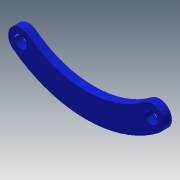
# Autodesk Inventor part: neco
Saved by Autodesk Inventor 2013 (Build 170138000, 138)
## iProperties
Created: 2013-03-09
Part Number: neco
Material: Generic
Document SubType Name: Modeling
Designer: idle-rug
Density: 1 g/cm^3
Author: idle-rug
Autodesk Inventor part; units mm, degrees
ref_plane "YZ Plane" through (0, 0, 0) normal (1, 0, 0) x (0, 1, 0)
ref_plane "XZ Plane" through (0, 0, 0) normal (0, 1, 0) x (-1, 0, 0)
ref_plane "XY Plane" through (0, 0, 0) normal (0, 0, 1) x (1, 0, 0)
sketch "Sketch1" plane through (0, 0, 0) normal (0, 1, 0) x (-1, 0, 0)
  line L0 (0, 0) -> (16, 0)
  line L1 (0, 0) -> (-16, 0)
  circle A0 centre (16, 0) radius 1.5
  circle A1 centre (-16, 0) radius 1.5
  circle A2 centre (16, 0) radius 3
  circle A3 centre (-16, 0) radius 3
  line L2 (14.1819, 2.3863) -> (16, 0)
  line L3 (16, 0) -> (17.8181, -2.3863)
  line L4 (-14.1819, 2.3863) -> (-16, 0)
  line L5 (-16, 0) -> (-17.8181, -2.3863)
  line L6 (0, -2.4008) -> (0, -8.4008)
  arc A4 (-17.8181, -2.3863) -> (17.8181, -2.3863) centre (0, 21) ccw
  arc A5 (-14.1819, 2.3863) -> (14.1819, 2.3863) centre (0, 21) ccw
  dimension "d2" = 3
  dimension "d11" = 6
  constraints: 14 end point, 10 point on circle, 6 centre point, 4 coincident, 3 collinear, 1 horizontal
  measures "d2" diameter of A0
  measures "d11" distance of L6.start L6.end
extrude "Extrusion1" add sketch "Sketch1" along normal blind 2 contours A5 A2 L0 | L0 A2 A4 L6 A5 | A5 L6 A4 A3 L1 | L1 A3 A5 | A2 L2 A0 L0 | L0 A0 L3 A2 | A2 L3 A0 L2 | A3 L5 A1 L1 | L1 A1 L4 A3 | L4 A1 L5 A3 | A0 L2 L0 | L0 L3 A0 | A0 L3 L2 | A1 L5 L1 | L1 L4 A1 | L4 L5 A1
sketch "Sketch2" plane through (0, 2, 0) normal (0, 1, 0) x (1, 0, 0)
  arc A0 (-17.8181, 2.3863) -> (-14.1819, -2.3863) centre (-16, 0) ccw projected
  arc A1 (14.1819, -2.3863) -> (17.8181, 2.3863) centre (16, 0) ccw projected
  circle A2 centre (-16, 0) radius 1.5
  circle A3 centre (16, 0) radius 1.5
  point P0 (0, 0)
  dimension "d14" = 3
  dimension "d15" = 3
  constraints: 2 centre point, 2 coincident
  measures "d14" diameter of A2
  measures "d15" diameter of A3
extrude "Extrusion2" cut sketch "Sketch2" against normal blind 2
body "Solid1"
